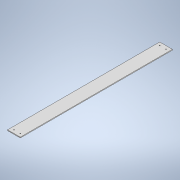
# Autodesk Inventor part: Flat Bar Drive
Saved by Autodesk Inventor 2020 (Build 240168000, 168)
## iProperties
Created: 2020-01-29
Part Number: Flat Bar Drive
Material: Generic
Document SubType Name: Modeling
Designer: aidan
Density: 1 g/cm^3
Appearance: Default
Author: aidan
Autodesk Inventor part; units mm, degrees
ref_plane "YZ Plane" through (0, 0, 0) normal (1, 0, 0) x (0, 1, 0)
ref_plane "XZ Plane" through (0, 0, 0) normal (0, 1, 0) x (-1, 0, 0)
ref_plane "XY Plane" through (0, 0, 0) normal (0, 0, 1) x (1, 0, 0)
sketch "Sketch1" plane through (0, 0, 0) normal (0, 0, 1) x (1, 0, 0)
  line L0 (-48.7274, 2.102) -> (2.0726, 2.102)
  line L1 (2.0726, 2.102) -> (2.0726, -1.073)
  line L2 (2.0726, -1.073) -> (-48.7274, -1.073)
  line L3 (-48.7274, -1.073) -> (-48.7274, 2.102)
  point P0 (0, 0)
  dimension "d0" = 3.175
  dimension "d1" = 50.8
  constraints: 8 end point, 2 parallel, 1 horizontal, 1 perpendicular
  measures "d0" distance of L0.end L1.end
  measures "d1" distance of L0.start L0.end
extrude "Extrusion1" add sketch "Sketch1" along normal blind 609.6
sketch "Sketch2" plane through (-48.7274, 2.102, 0) normal (0, 1, 0) x (1, 0, 0)
  circle A0 centre (12.7, -12.7) radius 1.7272
  circle A1 centre (38.1, -12.7) radius 1.7272
  line L0 (0, 0) -> (0, -609.6) projected
  line L1 (50.8, 0) -> (0, 0) projected
  line L2 (12.7, -12.7) -> (38.1, -12.7)
  point P0 (48.7274, 0)
  dimension "d5" = 3.4544
  dimension "d6" = 25.4
  dimension "d7" = 12.7
  dimension "d8" = 12.7
  constraints: 2 centre point, 2 end point, 1 equal radius, 1 horizontal
  measures "d5" diameter of A1
  measures "d6" distance of L2.end L2.start
  measures "d7" distance from line of L0 L2.start
  measures "d8" distance from line of L1 L2.start
extrude "Extrusion2" cut sketch "Sketch2" against normal through all
pattern_linear "Rectangular Pattern1" count 2 spacing 584.2 along (0, 0, 1) of "Extrusion2"
equation "\"d3\" = d2"
equation "\"d2\" = 609.6"
body "Solid1"
